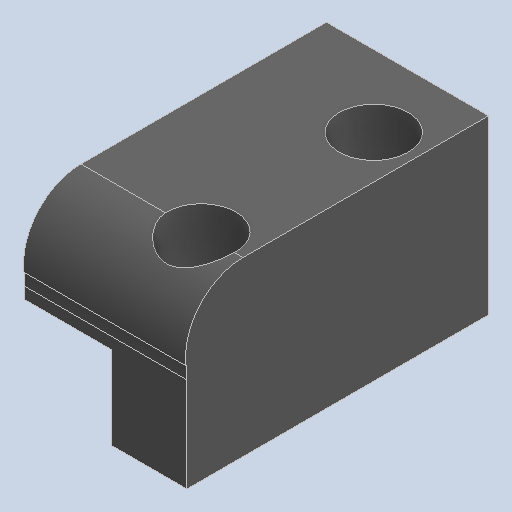
# Autodesk Inventor part: cam_setter_right_upper
Saved by Autodesk Inventor 2024.1 (Build 281209000, 209)
## iProperties
Created: 2025-03-04
Part Number: cam_setter_right_upper
Material: 一般
Document SubType Name: Modeling
Designer: hibik
Density: 1 g/cm^3
Appearance: 既定
Author: hibik
Autodesk Inventor part; units mm, degrees
ref_plane "YZ Plane" through (0, 0, 0) normal (1, 0, 0) x (0, 1, 0)
ref_plane "XZ Plane" through (0, 0, 0) normal (0, 1, 0) x (-1, 0, 0)
sketch "スケッチ1" plane through (0, 0, 0) normal (1, 0, 0) x (0, 1, 0)
  circle A0 centre (10, 5.37) radius 1.6
  circle A1 centre (10, -5.37) radius 1.6
  circle A2 centre (-10, -5.37) radius 1.6
  circle A3 centre (-10, 5.37) radius 1.6
  line L0 (-19.6, 0) -> (19.6, 0) projected
  line L1 (0, -13.118) -> (0, 13.118) projected
  line L2 (14, 9.37) -> (-14, 9.37)
  line L3 (-14, 9.37) -> (-14, -9.37)
  line L4 (-14, -9.37) -> (14, -9.37)
  line L5 (14, -9.37) -> (14, 9.37)
  point P0 (0, 0)
  dimension "d0" = 3.2
  dimension "d1" = 20
  dimension "d2" = 10.74
  dimension "d3" = 4
  dimension "d4" = 4
  constraints: 8 end point, 4 centre point, 3 equal radius, 2 horizontal alignment, 2 parallel, 2 symmetric about line, 2 vertical alignment, 1 horizontal, 1 perpendicular, 2 other
  measures "d0" diameter of A1
  measures "d1" distance of A3.centre A0.centre
  measures "d2" distance of A1.centre A0.centre
  measures "d3" distance from line of L4 A1.centre
  measures "d4" distance from line of L5 A1.centre
extrude "押し出し1" add sketch "スケッチ1" against normal blind 2
sketch "スケッチ2" plane through (0, 0, 0) normal (1, 0, 0) x (0, 0, -1)
  line L0 (9.37, 15.2) -> (-40.63, 15.2)
  line L1 (-40.63, 15.2) -> (-40.63, 0.2)
  line L2 (-40.63, 0.2) -> (9.37, 0.2)
  line L3 (9.37, 0.2) -> (9.37, 15.2)
  line L4 (9.37, -14) -> (9.37, 14) projected
  line L5 (9.37, 14) -> (-9.37, 14) projected
  circle A0 centre (-5.37, 10) radius 1.6 projected
  circle A1 centre (5.37, 10) radius 1.6 projected
  point P0 (0, 0)
  dimension "d7" = 1.2
  dimension "d8" = 50
  dimension "d9" = 15
  constraints: 8 end point, 2 parallel, 1 collinear, 1 horizontal, 1 perpendicular
  measures "d7" distance between parallel lines of L0 L5
  measures "d8" distance of L0.start L0.end
  measures "d9" distance of L0.end L1.end
extrude "押し出し2" add sketch "スケッチ2" against normal blind 6.6
sketch "スケッチ3" plane through (0, 15.2, 40.63) normal (0, 1, 0) x (1, 0, 0)
  line L0 (-6.6, 50) -> (-6.6, 0) projected
  line L1 (-6.6, 0) -> (0, 0)
  line L2 (0, 0) -> (0, 30)
  line L3 (0, 30) -> (-6.6, 30)
  line L4 (-6.6, 30) -> (-6.6, 0)
  line L5 (0, 50) -> (0, 0) projected
  point P0 (0, 40.63)
  dimension "d12" = 30
  constraints: 8 end point, 2 parallel, 1 collinear, 1 horizontal, 1 perpendicular
  measures "d12" distance between parallel lines of L1 L3
extrude "押し出し3" add sketch "スケッチ3" along normal blind 28
sketch "スケッチ4" plane through (-6.6, 0, 0) normal (-1, 0, 0) x (0, 0, 1)
  circle A0 centre (47.7718, 36.9277) radius 1.4 projected
  circle A1 centre (58.3718, 25.2) radius 1.4 projected
  circle A2 centre (55.0223, 40.3086) radius 1.4 projected
  circle A3 centre (50.3718, 25.2) radius 1.4 projected
  circle A4 centre (47.7718, 13.4723) radius 1.4 projected
  circle A5 centre (55.0223, 10.0914) radius 1.4 projected
  arc A6 (29.2731, 15.2) -> (26.2731, 15.2) centre (27.7731, 15.2) ccw projected
  line L0 (26.2731, 15.2) -> (16.4663, 15.2) projected
  arc A7 (16.4663, 35.2) -> (16.4663, 15.2) centre (32.6218, 25.2) ccw projected
  line L1 (16.4663, 35.2) -> (26.2731, 35.2) projected
  arc A8 (26.2731, 35.2) -> (29.2731, 35.2) centre (27.7731, 35.2) ccw projected
  line L2 (29.2731, 35.2) -> (36.8718, 35.2) projected
  line L3 (36.8718, 35.2) -> (36.8718, 36.2) projected
  arc A9 (44.8718, 44.2) -> (36.8718, 36.2) centre (44.8718, 36.2) ccw projected
  line L4 (44.8718, 44.2) -> (57.5369, 44.2) projected
  arc A10 (57.5369, 6.2) -> (57.5369, 44.2) centre (22.6218, 25.2) ccw projected
  line L5 (57.5369, 6.2) -> (44.8718, 6.2) projected
  arc A11 (36.8718, 14.2) -> (44.8718, 6.2) centre (44.8718, 14.2) ccw projected
  line L6 (36.8718, 14.2) -> (36.8718, 15.2) projected
  line L7 (36.8718, 15.2) -> (29.2731, 15.2) projected
  line L8 (-9.37, 0.2) -> (40.63, 0.2) projected
  line L9 (40.63, 0.2) -> (40.63, 43.2) projected
  line L10 (10.63, 43.2) -> (40.63, 43.2) projected
  line L11 (10.63, 15.2) -> (10.63, 43.2) projected
  line L12 (10.63, 15.2) -> (-9.37, 15.2) projected
  line L13 (-9.37, 15.2) -> (-9.37, 0.2) projected
  circle A12 centre (-5.37, 10) radius 1.6 projected
  circle A13 centre (5.37, 10) radius 1.6 projected
  line L14 (10.63, 15.2) -> (10.63, 0.2)
  line L15 (40.63, 42.9829) -> (10.63, 42.9829)
  point P0 (0, 0)
  point P1 (40.63, 7.4171)
  constraints: 4 end point, 3 point on line, 2 perpendicular, 1 point on circle
extrude "押し出し4" add sketch "スケッチ4" along normal blind 7.5 contours L7 L6 A11 L9 L8 L14 L11 L15 A9 L3 L2 A8 L1 A7 L0 A6
sketch "スケッチ5" plane through (-14.1, 0, 0) normal (-1, 0, 0) x (0, 0, 1)
  arc A0 (26.2731, 35.2) -> (29.2731, 35.2) centre (27.7731, 35.2) ccw projected
  arc A1 (29.2731, 15.2) -> (26.2731, 15.2) centre (27.7731, 15.2) ccw projected
  circle A2 centre (27.7731, 35.2) radius 1.25
  circle A3 centre (27.7731, 15.2) radius 1.25
  line L0 (26.2731, 35.2) -> (29.2731, 35.2)
  line L1 (29.2731, 15.2) -> (26.2731, 15.2)
  point P0 (0, 0)
  point P1 (26.5231, 15.2)
  point P2 (29.0231, 15.2)
  point P3 (29.0231, 35.2)
  point P4 (26.5231, 35.2)
  dimension "d17" = 2.5
  dimension "d18" = 2.5
  constraints: 4 end point, 2 centre point, 2 coincident, 1 horizontal, 1 parallel
  measures "d17" diameter of A2
  measures "d18" diameter of A3
extrude "押し出し5" cut sketch "スケッチ5" against normal up to surface (7.5 mm away) contours L0 A2 A0 | L1 A3 A1
sketch "スケッチ6" plane through (-14.1, 0, 0) normal (-1, 0, 0) x (0, 0, 1)
  line L0 (40.63, 0.2) -> (40.63, 7.4171) projected
  line L1 (40.63, 0.2) -> (20.63, 0.2)
  line L2 (20.63, 0.2) -> (20.63, 7.4171)
  line L3 (20.63, 7.4171) -> (40.63, 7.4171)
  line L4 (40.63, 7.4171) -> (40.63, 0.2)
  point P0 (0, 0)
  dimension "d22" = 20
  constraints: 8 end point, 2 parallel, 1 horizontal, 1 perpendicular, 1 point on line
  measures "d22" distance of L2.end L3.end
extrude "押し出し6" cut sketch "スケッチ6" against normal through all
fillet "フィレット2" radius 5 2 edges at (-10.35, 42.9829, 40.63) (-10.35, 7.4171, 40.63)
sketch "スケッチ7" plane through (-6.6, 0, 0) normal (-1, 0, 0) x (0, 0, 1)
  arc A0 (36.8718, 14.2) -> (36.9474, 13.1029) centre (44.8718, 14.2) ccw projected
  arc A1 (31.9946, 7.4171) -> (36.9474, 13.1029) centre (31.9946, 12.4171) ccw projected
  line L0 (31.9946, 7.4171) -> (40.63, 7.4171) projected
  line L1 (40.63, 7.4171) -> (40.63, 43.2) projected
  line L2 (10.63, 43.2) -> (40.63, 43.2) projected
  line L3 (10.63, 42.9829) -> (10.63, 43.2) projected
  line L4 (10.63, 42.9829) -> (31.9946, 42.9829) projected
  arc A2 (36.9474, 37.2971) -> (31.9946, 42.9829) centre (31.9946, 37.9829) ccw projected
  arc A3 (36.9474, 37.2971) -> (36.8718, 36.2) centre (44.8718, 36.2) ccw projected
  line L5 (36.8718, 36.2) -> (36.8718, 35.2) projected
  line L6 (36.8718, 35.2) -> (29.0231, 35.2) projected
  arc A4 (26.5231, 35.2) -> (29.0231, 35.2) centre (27.7731, 35.2) ccw projected
  line L7 (26.5231, 35.2) -> (16.4663, 35.2) projected
  arc A5 (16.4663, 35.2) -> (16.4663, 15.2) centre (32.6218, 25.2) ccw projected
  line L8 (16.4663, 15.2) -> (26.5231, 15.2) projected
  arc A6 (29.0231, 15.2) -> (26.5231, 15.2) centre (27.7731, 15.2) ccw projected
  line L9 (29.0231, 15.2) -> (36.8718, 15.2) projected
  line L10 (36.8718, 15.2) -> (36.8718, 14.2) projected
  line L11 (36.8718, 35.2) -> (36.8718, 15.2)
  point P0 (0, 0)
  constraints: 2 end point, 1 vertical
extrude "押し出し7" cut sketch "スケッチ7" against normal through all contours L10 L11 L5 A3 A2 L4 L3 L2 L1 L0 A1 A0
sketch "スケッチ8" plane through (0, 0, 0) normal (1, 0, 0) x (0, 0, -1)
  circle A0 centre (-19.37, 19.55) radius 1.6 projected
  circle A1 centre (-19.37, 19.55) radius 3.5
  point P0 (0, 0)
  dimension "d28" = 7
  constraints: 1 centre point, 1 coincident
  measures "d28" diameter of A1
extrude "押し出し8" cut sketch "スケッチ8" against normal through all contours A0 | A1
ref_plane "作業平面1" through (-14.1, 27.9829, 10.63) normal (0, 1, 0) x (1, 0, 0)
sketch "スケッチ9" plane through (-14.1, 27.9829, 10.63) normal (0, 1, 0) x (1, 0, 0)
  line L0 (42.7294, 46.3445) -> (-18.2888, 46.3445)
  line L1 (-18.2888, 46.3445) -> (-18.2888, -73.0893)
  line L2 (-18.2888, -73.0893) -> (42.7294, -73.0893)
  line L3 (42.7294, -73.0893) -> (42.7294, 46.3445)
  point P0 (14.1, 10.63)
  constraints: 8 end point, 2 parallel, 1 horizontal, 1 perpendicular
extrude "押し出し9" cut sketch "スケッチ9" against normal through all
sketch "スケッチ10" plane through (-14.1, 27.9829, 10.63) normal (0, -1, 0) x (1, 0, 0)
  circle A0 centre (10.35, 21.2418) radius 1.6 projected
  circle A1 centre (10.35, 6.2418) radius 1.6 projected
  point P0 (14.1, -10.63)
extrude "押し出し10" cut sketch "スケッチ10" against normal through all
sketch "スケッチ11" plane through (-14.1, 42.9829, 10.63) normal (0, 1, 0) x (1, 0, 0)
  circle A0 centre (10.35, -21.2418) radius 1.6 projected
  circle A1 centre (10.35, -6.2418) radius 1.6 projected
  circle A2 centre (10.35, -21.2418) radius 3
  circle A3 centre (10.35, -6.2418) radius 3
  point P0 (14.1, 10.63)
  dimension "d36" = 6
  dimension "d37" = 6
  constraints: 2 centre point, 2 coincident
  measures "d36" diameter of A2
  measures "d37" diameter of A3
extrude "押し出し11" cut sketch "スケッチ11" against normal blind 12 contours A1 | A2 | A3
fillet "フィレット3" radius 0.2 4 edges at (-6.6, 32.6343, 15.935) (-6.6, 33.0914, 17.8085) (-6.6, 33.0914, 32.8085) (-6.6, 33.0914, 30.935)
equation "\"d4\" = d3"
equation "\"d18\" = d17"
